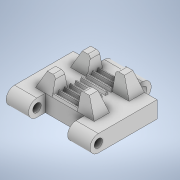
# Autodesk Inventor part: gasienica
Saved by Autodesk Inventor 2022 (Build 260153000, 153)
## iProperties
Created: 2022-04-02
Part Number: gasienica
Material: Ogólny
Document SubType Name: Modeling
Designer: jolow
Density: 1 g/cm^3
Appearance: Domyślna
Author: jolow
Autodesk Inventor part; units mm, degrees
ref_plane "YZ Plane" through (0, 0, 0) normal (1, 0, 0) x (0, 1, 0)
ref_plane "XZ Plane" through (0, 0, 0) normal (0, 1, 0) x (-1, 0, 0)
ref_plane "XY Plane" through (0, 0, 0) normal (0, 0, 1) x (1, 0, 0)
sketch "Szkic1" plane through (0, 0, 0) normal (0, 1, 0) x (-1, 0, 0)
  line L0 (0, 0) -> (30, 0)
  line L1 (30, 0) -> (30, 18)
  line L2 (30, 18) -> (0, 18)
  line L3 (0, 18) -> (0, 0)
  dimension "d0" = 18
  dimension "d1" = 30
  constraints: 8 end point, 2 parallel, 1 horizontal, 1 perpendicular
  measures "d0" distance of L0.end L1.end
  measures "d1" distance of L1.end L2.end
extrude "Wyciągnięcie proste1" add sketch "Szkic1" along normal blind 6
sketch "Szkic2" plane through (0, 6, 0) normal (0, 1, 0) x (1, 0, 0)
  line L0 (-30, -18) -> (0, -18) projected
  line L1 (0, -18) -> (-8, -18)
  line L2 (-8, -18) -> (-8, -24)
  line L3 (-8, -24) -> (0, -24)
  line L4 (0, -24) -> (0, -18)
  line L5 (-30, 0) -> (-30, -18) projected
  line L6 (-30, -18) -> (-22, -18)
  line L7 (-22, -18) -> (-22, -24)
  line L8 (-22, -24) -> (-30, -24)
  line L9 (-30, -24) -> (-30, -18)
  line L10 (0, 0) -> (-30, 0) projected
  line L11 (-15, 0) -> (-21.9, 0)
  line L12 (-21.9, 0) -> (-21.9, 6)
  line L13 (-21.9, 6) -> (-15, 6)
  line L14 (-15, 6) -> (-15, 0)
  line L15 (-15, 0) -> (-8.1, 0)
  line L16 (-8.1, 0) -> (-8.1, 6)
  line L17 (-8.1, 6) -> (-15, 6)
  line L18 (-15, 6) -> (-15, 0)
  dimension "d6" = 6
  dimension "d7" = 6
  dimension "d9" = 8
  dimension "d10" = 8
  dimension "d11" = 6
  dimension "d12" = 6.9
  dimension "d13" = 6.9
  dimension "d14" = 6
  constraints: 32 end point, 8 parallel, 4 horizontal, 4 perpendicular, 1 midpoint
  measures "d6" distance of L6.end L7.end
  measures "d7" distance of L3.end L0.end
  measures "d9" distance of L7.end L8.end
  measures "d10" distance of L2.end L3.end
  measures "d11" distance of L11.end L12.end
  measures "d12" distance of L12.end L13.end
  measures "d13" distance of L17.end L16.end
  measures "d14" distance of L15.end L16.end
extrude "Wyciągnięcie proste2" add sketch "Szkic2" against normal blind 6
sketch "Szkic3" plane through (0, 0, 0) normal (1, 0, 0) x (0, 0, -1)
  line L0 (-18, 0) -> (-18, 6) projected
  line L1 (-24, 6) -> (-24, 0) projected
  line L2 (0, 0) -> (-24, 0) projected
  line L3 (-24, 6) -> (0, 6) projected
  point P0 (-21, 3)
  dimension "d24" = 3
  dimension "d25" = 3
  dimension "d26" = 3
  dimension "d27" = 3
  measures "d24" distance from line of L0 point (-21, 3)
  measures "d25" distance from line of L1 point (-21, 3)
  measures "d26" distance from line of L2 point (-21, 3)
  measures "d27" distance from line of L3 point (-21, 3)
hole "Otwór1" at (0, 3, 21) direction (-1, 0, 0) diameter 3 end through all
fillet "Zaokrąglenie1" radius 3 2 edges at (-4, 6, 24) (-4, 0, 24)
fillet "Zaokrąglenie2" radius 3 4 edges at (-26, 0, 24) (-26, 6, 24) (-15, 6, -6) (-15, 0, -6)
sketch "Szkic4" plane through (-8.1, 0, 0) normal (1, 0, 0) x (0, 0, -1)
  line L0 (0, 0) -> (0, 6) projected
  point P0 (3, 3)
  point P1 (0, 3)
  point P2 (3, 0)
  constraints: 1 horizontal alignment, 1 midpoint, 1 vertical alignment
hole "Otwór2" at (-8.1, 3, -3) direction (-1, 0, 0) diameter 3 end through all
sketch "Szkic5" plane through (0, 6, 0) normal (0, 1, 0) x (1, 0, 0)
  line L0 (-22, -18) -> (-8, -18) projected
  line L1 (-19.5, -18) -> (-25.5, -18)
  line L2 (-25.5, -18) -> (-25.5, -12.5)
  line L3 (-25.5, -12.5) -> (-19.5, -12.5)
  line L4 (-19.5, -12.5) -> (-19.5, -18)
  line L5 (-10.5, -18) -> (-4.5, -18)
  line L6 (-4.5, -18) -> (-4.5, -12.5)
  line L7 (-4.5, -12.5) -> (-10.5, -12.5)
  line L8 (-10.5, -12.5) -> (-10.5, -18)
  line L9 (-10.5, 0) -> (-4.5, 0)
  line L10 (-4.5, 0) -> (-4.5, -5.5)
  line L11 (-4.5, -5.5) -> (-10.5, -5.5)
  line L12 (-10.5, -5.5) -> (-10.5, 0)
  line L13 (-19.5, 0) -> (-25.5, 0)
  line L14 (-25.5, 0) -> (-25.5, -5.5)
  line L15 (-25.5, -5.5) -> (-19.5, -5.5)
  line L16 (-19.5, -5.5) -> (-19.5, 0)
  line L17 (0, -21) -> (0, 0) projected
  line L18 (-30, 0) -> (-30, -21) projected
  dimension "d37" = 9
  dimension "d38" = 9
  dimension "d39" = 5.5
  dimension "d40" = 5.5
  dimension "d41" = 5.5
  dimension "d42" = 5.5
  dimension "d43" = 7
  dimension "d44" = 6
  dimension "d45" = 6
  dimension "d46" = 7
  dimension "d47" = 6
  dimension "d48" = 6
  dimension "d49" = 4.5
  dimension "d50" = 4.5
  constraints: 32 end point, 8 parallel, 6 point on line, 4 horizontal, 4 perpendicular
  measures "d37" distance between parallel lines of L8 L4
  measures "d38" distance between parallel lines of L12 L16
  measures "d39" distance of L5.end L6.end
  measures "d40" distance of L9.end L10.end
  measures "d41" distance of L15.end L13.start
  measures "d42" distance of L3.end L1.start
  measures "d43" distance between parallel lines of L7 L11
  measures "d44" distance of L2.end L3.end
  measures "d45" distance of L5.start L5.end
  measures "d46" distance between parallel lines of L15 L3
  measures "d47" distance of L10.end L11.end
  measures "d48" distance of L14.end L15.end
  measures "d49" distance between parallel lines of L17 L6
  measures "d50" distance between parallel lines of L18 L2
extrude "Wyciągnięcie proste3" add sketch "Szkic5" along normal blind 6
sketch "Szkic8" plane through (-4.5, 6, 5.5) normal (1, 0, 0) x (0, 0, -1)
  line L0 (0, 6) -> (5.5, 6) projected
  line L1 (0, 0) -> (0, 6) projected
  line L2 (1.2577, 6) -> (0, 0)
  point P0 (5.5, -6)
  constraints: 2 end point, 1 point on line
extrude "Wyciągnięcie proste4" cut sketch "Szkic8" against normal blind 60
sketch "Szkic9" plane through (-4.5, 6, 0) normal (1, 0, 0) x (0, 0, -1)
  line L0 (-4.2423, 6) -> (0, 6) projected
  line L1 (-1.2472, 6) -> (0, 0)
  line L2 (0, 6) -> (-4.2423, 6) projected
  line L3 (-1.2472, 6) -> (0, 6)
  line L4 (3, 0) -> (0, 0) projected
  line L5 (0, 6) -> (0, 0)
  point P0 (0, -6)
  constraints: 6 end point, 1 collinear, 1 perpendicular, 1 point on line
extrude "Wyciągnięcie proste5" cut sketch "Szkic9" against normal blind 60
sketch "Szkic13" plane through (0, 0, 0) normal (0, 0, 1) x (1, 0, 0)
  line L0 (-4.5, 6) -> (-7.5, 12.1595)
  line L1 (-4.5, 12) -> (-10.5, 12) projected
  line L2 (0, 6) -> (-4.5, 6) projected
  line L3 (-4.5, 12) -> (-4.5, 6) projected
  line L4 (-4.5, 6) -> (-4.5, 12)
  line L5 (-4.5, 6) -> (-4.5, 12.86)
  line L6 (-4.5, 12.86) -> (-7.8412, 12.86)
  line L7 (-7.8412, 12.86) -> (-7.5, 12.1595)
  point P0 (0, 0)
  point P1 (-7.4223, 12)
  constraints: 10 end point, 2 perpendicular, 1 vertical
extrude "Wyciągnięcie proste7" cut sketch "Szkic13" along normal blind 60 contours L0 L1 L3
sketch "Szkic14" plane through (-25.5, 6, 12.5) normal (-1, 0, 0) x (0, 0, 1)
  line L0 (0, 0) -> (0, 6) projected
  line L1 (0, 6) -> (1.25, 6)
  line L2 (0, 6) -> (5.5, 6) projected
  line L3 (1.25, 6) -> (4.25, 6)
  line L4 (4.25, 6) -> (5.5, 6)
  line L5 (0, 0) -> (5.5, 0) projected
  line L6 (1.25, 6) -> (0, 0)
  line L7 (0, 0) -> (0, 6)
  line L8 (5.5, -6) -> (5.5, 0) projected
  line L9 (4.25, 6) -> (5.5, 0)
  line L10 (5.5, 0) -> (5.5, 6)
  point P0 (-12.5, -6)
  dimension "d68" = 1.25
  dimension "d69" = 3
  dimension "d70" = 1.25
  constraints: 14 end point, 3 collinear, 2 point on line
  measures "d68" distance of L0.end L1.end
  measures "d69" distance of L1.end L3.end
  measures "d70" distance of L3.end L2.end
extrude "Wyciągnięcie proste8" cut sketch "Szkic14" against normal blind 60 contours L0 L1 L6 | L9 L2 L10
sketch "Szkic15" plane through (0, 0, 0) normal (0, 0, 1) x (1, 0, 0)
  line L0 (-19.5, 12) -> (-25.5, 12) projected
  line L1 (-25.5, 12) -> (-22.5, 12)
  line L2 (-25.5, 6) -> (-25.5, 12) projected
  line L3 (-22.5, 12) -> (-25.5, 6)
  line L4 (-25.5, 6) -> (-25.5, 12)
  point P0 (0, 0)
  dimension "d73" = 3
  constraints: 6 end point, 1 collinear, 1 midpoint
  measures "d73" distance of L0.end L1.end
extrude "Wyciągnięcie proste9" cut sketch "Szkic15" along normal blind 60
fillet "Zaokrąglenie3" radius 1 4 edges at (-10.5, 12, 2.7447) (-10.5, 12, 15.25) (-19.5, 12, 2.7447) (-19.5, 12, 15.25)
sketch "Szkic16" plane through (-10.5, 6, 12.5) normal (-1, 0, 0) x (0, 0, 1)
  line L0 (5.5, 0) -> (0, 0) projected
  line L1 (5.5, 0) -> (4.5, 0)
  line L2 (5.5, 0) -> (5, 1.5)
  line L3 (5, 1.5) -> (4.5, 0)
  point P0 (-12.5, -6)
  dimension "d77" = 1
  dimension "d83" = 1.5
  constraints: 6 end point, 1 equal length, 1 point on line
  measures "d77" distance of L0.start L1.end
  measures "d83" distance from line of L0 L2.end
extrude "Wyciągnięcie proste10" add sketch "Szkic16" along normal up to surface (9 mm away)
fillet "Zaokrąglenie4" radius 0.2 1 edges at (-15, 7.5, 17.5)
pattern_linear "Szyk prostokątny1" count 9 spacing 2 along (0, 0, -1) of "Zaokrąglenie4", "Wyciągnięcie proste10"
equation "\"d24\" = d25"
equation "\"d26\" = d27"
equation "\"d49\" = d50"
